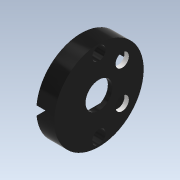
# Autodesk Inventor part: potentiometer_holder
Saved by Autodesk Inventor 2020.2 (Build 242310000, 310)
## iProperties
Created: 2020-05-03
Part Number: potentiometer_holder
Material: Generic
Document SubType Name: Modeling
Designer: Bardo91
Density: 1 g/cm^3
Appearance: Default
Author: Bardo91
Autodesk Inventor part; units mm, degrees
ref_plane "YZ Plane" through (0, 0, 0) normal (1, 0, 0) x (0, 1, 0)
ref_plane "XZ Plane" through (0, 0, 0) normal (0, 1, 0) x (-1, 0, 0)
ref_plane "XY Plane" through (0, 0, 0) normal (0, 0, 1) x (1, 0, 0)
sketch "Sketch1" plane through (0, 0, 0) normal (1, 0, 0) x (0, 1, 0)
  circle A0 centre (0, 0) radius 10
  line L0 (10, 0) -> (8.1, 0)
  circle A1 centre (8.1, 0) radius 1.5
  circle A2 centre (0, 0) radius 3
  circle A3 centre (-8.1, 0) radius 1.5
  dimension "d0" = 20
  dimension "d1" = 1.9
  dimension "d2" = 3
  dimension "d3" = 6
  dimension "d29" = 360
  constraints: 3 centre point, 3 coincident, 2 end point, 1 horizontal, 1 horizontal alignment, 7 other
  measures "d1" distance of L0.start L0.end
  measures "d2" diameter of A1
  measures "d3" diameter of A2
extrude "Extrusion1" add sketch "Sketch1" along normal blind 1
sketch "Sketch2" plane through (0, 0, 0) normal (-1, 0, 0) x (0, 0, 1)
  line L0 (0, 5.5) -> (-6.5, 5.5)
  line L1 (0, 5.5) -> (2.5, 5.5)
  line L2 (6.0478, 3.0122) -> (6.0478, -2.8019)
  line L3 (-6.5, -5.5) -> (-6.5, 5.5)
  line L4 (5.5, 5.498) -> (2.5, 5.5)
  line L5 (2.5, 5.5) -> (6.0478, 3.0122)
  line L6 (5.2, -5.498) -> (2.2, -5.5)
  line L7 (2.2, -5.5) -> (6.0478, -2.8019)
  line L8 (2.2, -5.5) -> (-6.5, -5.5)
  line L9 (2.5631, 5.7) -> (6.585, 2.8798)
  line L10 (6.585, 2.8798) -> (6.585, -2.7667)
  line L11 (6.585, -2.7667) -> (2.4018, -5.7)
  line L12 (2.5631, 5.7) -> (0, 5.7)
  line L13 (0, 5.7) -> (-6.7, 5.7)
  line L14 (-6.7, 5.7) -> (-6.7, -5.7)
  line L15 (-6.7, -5.7) -> (2.4018, -5.7)
  circle A0 centre (0, 0) radius 10
  circle A1 centre (0, 0) radius 10 projected
  line L16 (10, 0) -> (10, 1)
  line L17 (10, 1) -> (6.585, 1)
  line L18 (10, 0) -> (10, -1)
  line L19 (10, 0) -> (11, 0) construction
  line L20 (10, -1) -> (6.585, -1)
  line L21 (-10, 0) -> (-10, 3.5)
  line L22 (-10, 3.5) -> (-6.7, 3.5)
  line L23 (-10, 0) -> (-10, -3.5)
  line L24 (-10, -3.5) -> (-6.7, -3.5)
  circle A2 centre (0, 8.1) radius 1.5 projected
  circle A3 centre (0, 8.1) radius 1.5
  circle A4 centre (0, -8.1) radius 1.5
  point P0 (-9.3675, -3.5)
  point P1 (9.9499, -1)
  point P2 (9.9499, 1)
  point P3 (-9.3675, 3.5)
  dimension "d6" = 5.5
  dimension "d7" = 6.5
  dimension "d8" = 5.5
  dimension "d9" = 11
  dimension "d10" = 3
  dimension "d11" = 35
  dimension "d12" = 3
  dimension "d13" = 35
  dimension "d14" = 0.2
  dimension "d15" = 0.2
  dimension "d18" = 1
  dimension "d19" = 1
  dimension "d20" = 270
  dimension "d21" = 3.5
  dimension "d22" = 3.5
  dimension "d33" = 360
  constraints: 50 end point, 11 perpendicular, 6 point on line, 5 horizontal, 3 centre point, 3 tangent, 2 coincident, 2 point on circle, 1 parallel, 1 vertical, 6 other
  measures "d6" distance of point (0, 0) L0.start
  measures "d7" distance of L0.start L0.end
  measures "d8" distance of L0.start L4.start
  measures "d9" distance of L4.start L6.start
  measures "d10" distance of L1.end L4.start
  measures "d11" angle of L5 L4
  measures "d12" distance of L6.start L6.end
  measures "d13" angle of L6 L7
  measures "d14" distance between parallel lines of L5 L9
  measures "d15" distance between parallel lines of L1 L12
  measures "d18" distance of L16.start L16.end
  measures "d19" distance of L16.start L18.end
  measures "d21" distance of L21.start L21.end
  measures "d22" distance of L21.start L23.end
extrude "Extrusion2" add sketch "Sketch2" along normal blind 3 contours L9 L12 L13 L14 L22 A0 L17 L10 | L11 L10 L20 A0 L24 L14 L15
sketch "Sketch3" plane through (0, 0, 0) normal (-1, 0, 0) x (0, 0, 1)
  circle A0 centre (-5.2, 4.2) radius 1.5
  circle A1 centre (-5.2, -4.2) radius 1.5
  line L0 (-6.7, 5.7) -> (2.5631, 5.7) projected
  line L1 (-6.7, 3.5) -> (-6.7, 5.7) projected
  line L2 (-6.7, -5.7) -> (-6.7, -3.5) projected
  line L3 (2.4018, -5.7) -> (-6.7, -5.7) projected
  point P0 (0, 0)
  dimension "d23" = 3
  dimension "d24" = 3
  constraints: 4 tangent, 2 centre point
  measures "d23" diameter of A0
  measures "d24" diameter of A1
extrude "Extrusion3" cut sketch "Sketch3" against normal blind 10 contours A0 | A1
body "Solid1"
